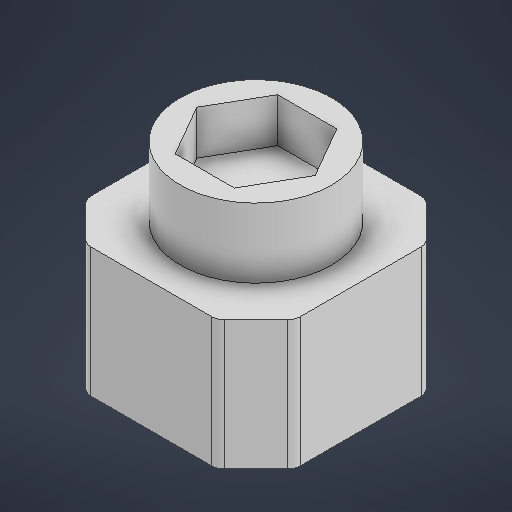
# Autodesk Inventor part: newAdapter
Saved by Autodesk Inventor 2026 (Build 300175050, 175E)
## iProperties
Created: 2025-10-28
Part Number: newAdapter
Material: Generic
Document SubType Name: Modeling
Designer: aduwa
Density: 1 g/cm^3
Appearance: Default
Author: aduwa
Autodesk Inventor part; units mm, degrees
ref_plane "YZ Plane" through (0, 0, 0) normal (1, 0, 0) x (0, 1, 0)
ref_plane "XZ Plane" through (0, 0, 0) normal (0, 1, 0) x (-1, 0, 0)
ref_plane "XY Plane" through (0, 0, 0) normal (0, 0, 1) x (1, 0, 0)
sketch "Sketch1" plane through (0, 0, 0) normal (0, 1, 0) x (-1, 0, 0)
  circle A0 centre (0, 0) radius 6
  line L0 (5.2886, 8.5) -> (-5.2886, 8.5)
  line L1 (-8.5, 5.2886) -> (-8.5, -5.2886)
  line L2 (-5.2886, -8.5) -> (5.2886, -8.5)
  line L3 (8.5, -5.2886) -> (8.5, 5.2886)
  line L4 (8.5, 8.5) -> (-8.5, -8.5) construction
  line L5 (-8.5, 8.5) -> (8.5, -8.5) construction
  line L6 (-6.8943, -6.8943) -> (6.8943, 6.8943)
  line L7 (8.5, 5.2886) -> (5.2886, 8.5)
  line L8 (-5.2886, -8.5) -> (-8.5, -5.2886)
  line L9 (0, 0) -> (2.4857, 0)
  line L10 (8.5, -5.2886) -> (5.2886, -8.5)
  line L11 (-5.2886, 8.5) -> (-8.5, 5.2886)
  line L12 (8.3, 5.2057) -> (8.3, -5.2057)
  line L13 (8.3, -5.2057) -> (5.2057, -8.3)
  line L14 (5.2057, -8.3) -> (-5.2057, -8.3)
  line L15 (-5.2057, -8.3) -> (-8.3, -5.2057)
  line L16 (-8.3, -5.2057) -> (-8.3, 5.2057)
  line L17 (-8.3, 5.2057) -> (-5.2057, 8.3)
  line L18 (-5.2057, 8.3) -> (5.2057, 8.3)
  line L19 (5.2057, 8.3) -> (8.3, 5.2057)
  dimension "d0" = 12
  dimension "d2" = 17
  dimension "d3" = 19.5
  dimension "d4" = 17
  dimension "d5" = 0.2
  constraints: 40 end point, 6 parallel, 5 midpoint, 4 symmetric about line, 2 horizontal, 2 perpendicular, 1 centre point, 1 coincident, 1 point on line, 7 other
  measures "d0" diameter of A0
  measures "d2" distance of L4.end L5.start
  measures "d3" distance of L6.start L6.end
  measures "d4" distance between parallel lines of L1 L3
  measures "d5" distance between parallel lines of L3 L12
extrude "Extrusion1" add sketch "Sketch1" along normal blind 10.25 contours A0 L6 L19 L12 L13 L14 L15 | A0 L6 L15 L16 L17 L18 L19
fillet "Fillet1" radius 1 8 edges at (-5.2057, 5.125, 8.3) (5.2057, 5.125, 8.3) (8.3, 5.125, 5.2057) (8.3, 5.125, -5.2057) (5.2057, 5.125, -8.3) (-5.2057, 5.125, -8.3) (-8.3, 5.125, 5.2057) (-8.3, 5.125, -5.2057)
sketch "Sketch2" plane through (0, 10.25, 0) normal (0, 1, 0) x (1, 0, 0)
  line L0 (4.5207, 0) -> (2.2603, -3.915)
  line L1 (2.2603, -3.915) -> (-2.2603, -3.915)
  line L2 (-2.2603, -3.915) -> (-4.5207, 0)
  line L3 (-4.5207, 0) -> (-2.2603, 3.915)
  line L4 (-2.2603, 3.915) -> (2.2603, 3.915)
  line L5 (2.2603, 3.915) -> (4.5207, 0)
  line L6 (2.3469, -4.065) -> (4.6939, 0)
  line L7 (4.6939, 0) -> (2.3469, 4.065)
  line L8 (2.3469, 4.065) -> (-2.3469, 4.065)
  line L9 (-2.3469, 4.065) -> (-4.6939, 0)
  line L10 (-4.6939, 0) -> (-2.3469, -4.065)
  line L11 (-2.3469, -4.065) -> (2.3469, -4.065)
  circle A0 centre (0, 0) radius 3.5
  arc A1 (-8.0071, 5.4986) -> (-8.3, 4.7915) centre (-7.3, 4.7915) ccw projected
  line L12 (-8.3, 4.7915) -> (-8.3, -4.7915) projected
  arc A2 (-8.3, -4.7915) -> (-8.0071, -5.4986) centre (-7.3, -4.7915) ccw projected
  line L13 (-8.0071, -5.4986) -> (-5.4986, -8.0071) projected
  arc A3 (-5.4986, -8.0071) -> (-4.7915, -8.3) centre (-4.7915, -7.3) ccw projected
  line L14 (-4.7915, -8.3) -> (4.7915, -8.3) projected
  arc A4 (4.7915, -8.3) -> (5.4986, -8.0071) centre (4.7915, -7.3) ccw projected
  line L15 (5.4986, -8.0071) -> (8.0071, -5.4986) projected
  arc A5 (8.0071, -5.4986) -> (8.3, -4.7915) centre (7.3, -4.7915) ccw projected
  line L16 (8.3, -4.7915) -> (8.3, 4.7915) projected
  arc A6 (8.3, 4.7915) -> (8.0071, 5.4986) centre (7.3, 4.7915) ccw projected
  line L17 (8.0071, 5.4986) -> (5.4986, 8.0071) projected
  arc A7 (5.4986, 8.0071) -> (4.7915, 8.3) centre (4.7915, 7.3) ccw projected
  line L18 (4.7915, 8.3) -> (-4.7915, 8.3) projected
  arc A8 (-4.7915, 8.3) -> (-5.4986, 8.0071) centre (-4.7915, 7.3) ccw projected
  line L19 (-5.4986, 8.0071) -> (-8.0071, 5.4986) projected
  circle A9 centre (0, 0) radius 6 projected
  dimension "d9" = 7.83
  dimension "d10" = 0.15
  dimension "d11" = 7
  constraints: 24 end point, 2 coincident, 1 centre point, 18 other
  measures "d9" distance between parallel lines of L4 L1
  measures "d10" distance between parallel lines of L0 L6
  measures "d11" diameter of A0
extrude "Extrusion2" add sketch "Sketch2" along normal blind 5.5 contours A9
extrude "Extrusion3" add sketch "Sketch2" along normal blind 2 contours L0 L1 L2 L3 L4 L5 | L11 L10 L9 L8 L7 L6 | A0
body "Solid1"
